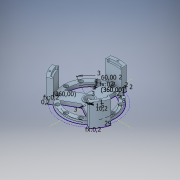
# Autodesk Inventor part: Enclosure2
Saved by Autodesk Inventor 2018.3 (Build 223284000, 284)
## iProperties
Created: 2018-07-23
Part Number: Enclosure2
Material: Generisch
Document SubType Name: Modeling
Designer: JochenAlt
Density: 1 g/cm^3
Appearance: Vorgabe
Author: JochenAlt
Autodesk Inventor part; units mm, degrees
ref_plane "YZ Plane" through (0, 0, 0) normal (1, 0, 0) x (0, 1, 0)
ref_plane "XZ Plane" through (0, 0, 0) normal (0, 1, 0) x (-1, 0, 0)
ref_plane "XY Plane" through (0, 0, 0) normal (0, 0, 1) x (1, 0, 0)
sketch "Skizze1" plane through (0, 0, 0) normal (0, 0, 1) x (1, 0, 0)
  circle A0 centre (0, 0) radius 29 construction
  circle A1 centre (0, 0) radius 5.1
  circle A2 centre (0, 0) radius 6.6
  circle A3 centre (0, 0) radius 4.1
  line L0 (0, 52.8) -> (0, -50.8) construction
  line L1 (-53.0726, 0) -> (53.0726, 0) construction
  line L2 (-8, 24.7386) -> (-8, 5.3066)
  line L3 (0, 0) -> (-28.9685, 16.725) construction
  line L4 (-25.4243, -5.4411) -> (-8.5957, 4.2749)
  arc A4 (-8, 5.3066) -> (-8.5957, 4.2749) centre (0, 0) ccw
  arc A5 (-8, 24.7386) -> (-25.4243, -5.4411) centre (0, 0) ccw
  line L5 (17.4243, -19.2975) -> (0.5957, -9.5815)
  arc A6 (-17.4243, -19.2975) -> (17.4243, -19.2975) centre (0, 0) ccw
  line L6 (-17.4243, -19.2975) -> (-0.5957, -9.5815)
  arc A7 (-0.5957, -9.5815) -> (0.5957, -9.5815) centre (0, 0) ccw
  line L7 (8, 24.7386) -> (8, 5.3066)
  arc A8 (25.4243, -5.4411) -> (8, 24.7386) centre (0, 0) ccw
  line L8 (25.4243, -5.4411) -> (8.5957, 4.2749)
  arc A9 (8.5957, 4.2749) -> (8, 5.3066) centre (0, 0) ccw
  circle A10 centre (0, 29) radius 2.1
  circle A11 centre (-14.5, 25.1147) radius 2.1
  circle A12 centre (-25.1147, 14.5) radius 2.1
  circle A13 centre (-29, 0) radius 2.1
  circle A14 centre (-25.1147, -14.5) radius 2.1
  circle A15 centre (-14.5, -25.1147) radius 2.1
  circle A16 centre (0, -29) radius 2.1
  circle A17 centre (14.5, -25.1147) radius 2.1
  circle A18 centre (25.1147, -14.5) radius 2.1
  circle A19 centre (29, 0) radius 2.1
  circle A20 centre (25.1147, 14.5) radius 2.1
  circle A21 centre (0, 0) radius 32
  circle A22 centre (14.5, 25.1147) radius 2.1
  line L9 (-8, 30.9839) -> (-8, 37.1484)
  line L10 (8, 30.9839) -> (8, 37.1484)
  line L11 (-30.8328, -8.5637) -> (-36.1714, -11.646)
  line L12 (22.8328, -22.4201) -> (28.1714, -25.5024)
  line L13 (30.8328, -8.5637) -> (36.1714, -11.646)
  line L14 (-22.8328, -22.4201) -> (-28.1714, -25.5024)
  arc A23 (8, 33.0454) -> (-8, 33.0454) centre (0, 0) ccw
  arc A24 (-32.6182, -9.5945) -> (-24.6182, -23.4509) centre (0, 0) ccw
  arc A25 (24.6182, -23.4509) -> (32.6182, -9.5945) centre (0, 0) ccw
  line L15 (-31.3249, -6.5384) -> (-36.749, -9.67)
  line L16 (-21.3249, -23.8589) -> (-26.749, -26.9906)
  line L17 (-10, 30.3974) -> (-10, 36.6606)
  line L18 (10, 30.3974) -> (10, 36.6606)
  line L19 (21.3249, -23.8589) -> (26.749, -26.9906)
  line L20 (31.3249, -6.5384) -> (36.749, -9.67)
  arc A26 (10, 36.6606) -> (-10, 36.6606) centre (0, 0) ccw
  arc A27 (-36.749, -9.67) -> (-26.749, -26.9906) centre (0, 0) ccw
  arc A28 (26.749, -26.9906) -> (36.749, -9.67) centre (0, 0) ccw
  line L21 (-25.1147, -14.5) -> (0, 0) construction
  circle A29 centre (0, 29) radius 2
  circle A30 centre (14.5, 25.1147) radius 2
  circle A31 centre (25.1147, 14.5) radius 2
  circle A32 centre (29, 0) radius 2
  circle A33 centre (25.1147, -14.5) radius 2
  circle A34 centre (14.5, -25.1147) radius 2
  circle A35 centre (0, -29) radius 2
  circle A36 centre (-14.5, -25.1147) radius 2
  circle A37 centre (-25.1147, -14.5) radius 2
  circle A38 centre (-29, 0) radius 2
  circle A39 centre (-25.1147, 14.5) radius 2
  circle A40 centre (-14.5, 25.1147) radius 2
  line L22 (-32.3816, -9.6888) -> (-30.7769, -8.7624)
  line L23 (-24.5816, -23.1988) -> (-22.9769, -22.2724)
  arc A41 (-32.3816, -9.6888) -> (-24.5816, -23.1988) centre (0, 0) ccw
  arc A42 (24.5816, -23.1988) -> (32.3816, -9.6888) centre (0, 0) ccw
  line L24 (32.3816, -9.6888) -> (30.7769, -8.7624)
  line L25 (24.5816, -23.1988) -> (22.9769, -22.2724)
  arc A43 (7.8, 32.8877) -> (-7.8, 32.8877) centre (0, 0) ccw
  line L26 (-7.8, 32.8877) -> (-7.8, 31.0348)
  line L27 (7.8, 32.8877) -> (7.8, 31.0348)
  circle A44 centre (0, 36) radius 1
  circle A45 centre (0, 0) radius 36 construction
  circle A46 centre (31.1769, -18) radius 1
  circle A47 centre (-31.1769, -18) radius 1
  point P0 (0, -9.6)
  dimension "d1" = 29
  dimension "d2" = 10.2
  dimension "d12" = 1
  dimension "d17" = 60
  dimension "d20" = 8
  dimension "d23" = 360
  dimension "d32" = 360
  dimension "d35" = 3
  dimension "d36" = 3
  dimension "d41" = 2
  dimension "d43" = 4
  dimension "d44" = 2
  dimension "d63" = 1.5
  dimension "d66" = 3
  dimension "d67" = 2.1
  dimension "d68" = 4
  dimension "d71" = 360
  dimension "d75" = 0.2
  dimension "d76" = 0.2
  dimension "d79" = 0.2
  dimension "d80" = 0.2
  dimension "d81" = 2
  dimension "d82" = 2
  constraints: 52 end point, 47 centre point, 42 point on circle, 13 coincident, 11 point on line, 8 equal radius, 6 collinear, 5 parallel, 3 vertical, 2 midpoint, 119 other
  measures "d1" radius of A0
  measures "d2" diameter of A1
  measures "d12" radial gap between concentric circles of A1 A3
  measures "d17" angle of L0 L3
  measures "d20" distance between parallel lines of L0 L2
  measures "d35" radial gap between concentric circles of A5 A0
  measures "d43" radial gap between concentric circles of A26 A23
  measures "d44" distance between parallel lines of L17 L9
  measures "d63" radial gap between concentric circles of A2 A1
  measures "d66" radial gap between concentric circles of A7 A2
  measures "d67" radius of A10
  measures "d68" diameter of A29
  measures "d75" distance between parallel lines of L14 L23
  measures "d76" radial gap between concentric circles of A24 A41
  measures "d79" distance between parallel lines of L9 L26
  measures "d80" distance between parallel lines of L12 L25
  measures "d81" diameter of A44
  measures "d82" radial gap between concentric circles of A45 A23
extrude "Extrusion1" add sketch "Skizze1" along normal blind 1.5 contours A1 | A2 | A10 | A11 | A12 | A13 | A14 | A15 | A16 | A17 | A18 | A19 | A20 | A21 | A21 L10 A26 L18 | L20 A28 L13 A21 | A21 L27 A43 L26 L9 A23 L10 | L13 A25 L12 A21 L25 A42 L24 | A21 L26 A43 L27 | A23 L9 A26 L10 | L24 A42 L25 A21 | L13 A28 L12 A25 | L9 A21 L17 A26 | L12 A28 L19 A21 | A21 L11 A27 L15 | L16 A27 L14 A21 | A21 L22 A41 L23 L14 A24 L11 | A21 L23 A41 L22 | A24 L14 A27 L11 | A22 | A29 | A30 | A31 | A32 | A33 | A34 | A35 | A36 | A37 | A38 | A39 | A40
extrude "Extrusion2" add sketch "Skizze1" along normal blind 3 from surface at 1.5 contours A2 | A21 | A21 L10 A26 L18 | L20 A28 L13 A21 | A21 L27 A43 L26 L9 A23 L10 | L13 A25 L12 A21 L25 A42 L24 | A21 L26 A43 L27 | A23 L9 A26 L10 | L24 A42 L25 A21 | L13 A28 L12 A25 | L9 A21 L17 A26 | L12 A28 L19 A21 | A21 L11 A27 L15 | L16 A27 L14 A21 | A21 L22 A41 L23 L14 A24 L11 | A21 L23 A41 L22 | A24 L14 A27 L11
extrude "Extrusion12" add sketch "Skizze1" along normal blind 1 from surface at 4.5 contours A2
extrude "Extrusion6" add sketch "Skizze1" along normal blind 21 from surface at 4.5 contours A21 L10 A26 L18 | L20 A28 L13 A21 | A21 L27 A43 L26 L9 A23 L10 | L13 A25 L12 A21 L25 A42 L24 | A21 L26 A43 L27 | A23 L9 A26 L10 | L24 A42 L25 A21 | L13 A28 L12 A25 | L9 A21 L17 A26 | L12 A28 L19 A21 | A21 L11 A27 L15 | L16 A27 L14 A21 | A21 L22 A41 L23 L14 A24 L11 | A21 L23 A41 L22 | A24 L14 A27 L11
chamfer "Fase1" distance 0.5 angle 45 12 edges at (-27.2147, -14.5, 4.5) (-31.1, 0, 4.5) (-27.2147, 14.5, 4.5) (-16.6, 25.1147, 4.5) (-2.1, 29, 4.5) (12.4, 25.1147, 4.5) (23.0147, 14.5, 4.5) (26.9, 0, 4.5) (-16.6, -25.1147, 4.5) (-2.1, -29, 4.5) (12.4, -25.1147, 4.5) (23.0147, -14.5, 4.5)
extrude "Extrusion7" add sketch "Skizze1" along normal blind 3 from surface at 25.5 contours A21 L10 A26 L18 | L20 A28 L13 A21 | A23 L9 A26 L10 | L13 A28 L12 A25 | L9 A21 L17 A26 | L12 A28 L19 A21 | A21 L11 A27 L15 | L16 A27 L14 A21 | A24 L14 A27 L11
